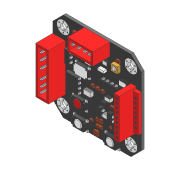
# Autodesk Inventor part: Closed Loop Driver Nema 17
Saved by Autodesk Inventor 2022 (Build 260153000, 153)
## iProperties
Created: 2024-03-01
Part Number: Closed Loop Driver Nema 17
Material: Generic
Document SubType Name: Modeling
Designer: jeffz
Mass: 3.6094 g
Surface Area: 65.104 cm^2
Volume: 3.6094 cm^3
Density: 1 g/cm^3
Appearance: Default
Author: jeffz
Autodesk Inventor part; units mm, degrees
(part 1 of 2)
ref_plane "YZ Plane" through (0, 0, 0) normal (1, 0, 0) x (0, 1, 0)
ref_plane "XZ Plane" through (0, 0, 0) normal (0, 1, 0) x (-1, 0, 0)
ref_plane "XY Plane" through (0, 0, 0) normal (0, 0, 1) x (1, 0, 0)
sketch "Sketch1" plane through (0, 0, 0) normal (0, 0, 1) x (1, 0, 0)
  line L0 (-16, -21) -> (16, -21)
  line L1 (21, -16) -> (21, 16)
  line L2 (16, 21) -> (-16, 21)
  line L3 (-21, 16) -> (-21, -16)
  circle A0 centre (16, 16) radius 1.5
  line L4 (16, 21) -> (21, 16)
  circle A1 centre (16, -16) radius 1.5
  line L5 (21, -16) -> (16, -21)
  circle A2 centre (-16, -16) radius 1.5
  line L6 (-16, -21) -> (-21, -16)
  circle A3 centre (-16, 16) radius 1.5
  line L7 (-21, 16) -> (-16, 21)
  point P0 (0, 0)
  dimension "d2" = 360
  constraints: 16 end point, 4 centre point, 2 parallel, 1 horizontal, 1 perpendicular, 21 other
extrude "Extrusion1" add sketch "Sketch1" along normal blind 1.25
sketch "Sketch2" plane through (0, 0, 1.25) normal (0, 0, 1) x (1, 0, 0)
  circle A0 centre (-16, 16) radius 1.5 projected
  circle A1 centre (-16, -16) radius 1.5 projected
  circle A2 centre (16, -16) radius 1.5 projected
  circle A3 centre (16, 16) radius 1.5 projected
  circle A4 centre (-16, 16) radius 3
  circle A5 centre (-16, 18.2261) radius 0.25
  circle A6 centre (-17.9279, 17.1131) radius 0.25
  circle A7 centre (-17.9279, 14.8869) radius 0.25
  circle A8 centre (-16, 13.7739) radius 0.25
  circle A9 centre (-14.0721, 14.8869) radius 0.25
  circle A10 centre (-14.0721, 17.1131) radius 0.25
  circle A11 centre (-16, -16) radius 3
  circle A12 centre (-16, -13.7739) radius 0.25
  circle A13 centre (-17.9279, -14.8869) radius 0.25
  circle A14 centre (-17.9279, -17.1131) radius 0.25
  circle A15 centre (-16, -18.2261) radius 0.25
  circle A16 centre (-14.0721, -17.1131) radius 0.25
  circle A17 centre (-14.0721, -14.8869) radius 0.25
  circle A18 centre (16, -16) radius 3
  circle A19 centre (16, -13.7739) radius 0.25
  circle A20 centre (14.0721, -14.8869) radius 0.25
  circle A21 centre (14.0721, -17.1131) radius 0.25
  circle A22 centre (16, -18.2261) radius 0.25
  circle A23 centre (17.9279, -17.1131) radius 0.25
  circle A24 centre (17.9279, -14.8869) radius 0.25
  circle A25 centre (16, 16) radius 3
  circle A26 centre (16, 18.2261) radius 0.25
  circle A27 centre (14.0721, 17.1131) radius 0.25
  circle A28 centre (14.0721, 14.8869) radius 0.25
  circle A29 centre (16, 13.7739) radius 0.25
  circle A30 centre (17.9279, 14.8869) radius 0.25
  circle A31 centre (17.9279, 17.1131) radius 0.25
  point P0 (0, 0)
  dimension "d8" = 360
  dimension "d12" = 360
  dimension "d17" = 360
  dimension "d24" = 360
  constraints: 28 centre point, 52 other
extrude "Extrusion2" add sketch "Sketch2" along normal blind 0.05
sketch "Sketch3" plane through (0, 0, 1.25) normal (0, 0, 1) x (1, 0, 0)
  line L0 (-16, -21) -> (16, -21) projected
  line L1 (21, -16) -> (21, 16) projected
  line L2 (16, 21) -> (-16, 21) projected
  line L3 (-21, 16) -> (-21, -16) projected
  line L4 (-21, 11) -> (-15, 11)
  line L5 (-15, 11) -> (-15, -11)
  line L6 (-15, -11) -> (-21, -11)
  line L7 (-21, -11) -> (-21, 11)
  line L8 (-6, 21) -> (6, 21)
  line L9 (6, 21) -> (6, 15)
  line L10 (6, 15) -> (-6, 15)
  line L11 (-6, 15) -> (-6, 21)
  line L12 (18.5, 9) -> (16, 9)
  line L13 (16, 9) -> (16, -10)
  line L14 (16, -10) -> (18.5, -10)
  line L15 (18.5, -10) -> (18.5, 9)
  line L16 (-11, 14) -> (-8, 14)
  line L17 (-8, 14) -> (-8, 11)
  line L18 (-8, 11) -> (-11, 11)
  line L19 (-11, 11) -> (-11, 14)
  line L20 (8, 14) -> (11, 14)
  line L21 (11, 14) -> (11, 11)
  line L22 (11, 11) -> (8, 11)
  line L23 (8, 11) -> (8, 14)
  line L24 (-11, -21) -> (-4, -21)
  line L25 (-4, -21) -> (-4, -16)
  line L26 (-4, -16) -> (-11, -16)
  line L27 (-11, -16) -> (-11, -21)
  line L28 (4, -21) -> (11, -21)
  line L29 (11, -21) -> (11, -16)
  line L30 (11, -16) -> (4, -16)
  line L31 (4, -16) -> (4, -21)
  line L32 (-11.3467, -13) -> (-4.3467, -13)
  line L33 (-4.3467, -13) -> (-4.3467, -8)
  line L34 (-4.3467, -8) -> (-11.3467, -8)
  line L35 (-11.3467, -8) -> (-11.3467, -13)
  line L36 (-10, 1) -> (-3, 1)
  line L37 (-3, 1) -> (-3, 6)
  line L38 (-3, 6) -> (-10, 6)
  line L39 (-10, 6) -> (-10, 1)
  line L40 (-13, 0) -> (-13, -7)
  line L41 (-13, -7) -> (-8, -7)
  line L42 (-8, -7) -> (-8, 0)
  line L43 (-8, 0) -> (-13, 0)
  line L44 (11.7259, -10) -> (15, -10)
  line L45 (15, -10) -> (15, -12)
  line L46 (15, -12) -> (11.7259, -12)
  line L47 (11.7259, -12) -> (11.7259, -10)
  line L48 (11.7259, 9) -> (15, 9)
  line L49 (15, 9) -> (15, 7)
  line L50 (15, 7) -> (11.7259, 7)
  line L51 (11.7259, 7) -> (11.7259, 9)
  line L52 (-6, 13.2927) -> (-4.3467, 13.2927)
  line L53 (-4.3467, 13.2927) -> (-4.3467, 11.7259)
  line L54 (-4.3467, 11.7259) -> (-6, 11.7259)
  line L55 (-6, 11.7259) -> (-6, 13.2927)
  line L56 (-3, 13.2927) -> (-1.3141, 13.2927)
  line L57 (-1.3141, 13.2927) -> (-1.3141, 11.7259)
  line L58 (-1.3141, 11.7259) -> (-3, 11.7259)
  line L59 (-3, 11.7259) -> (-3, 13.2927)
  line L60 (1, 13.2927) -> (2.426, 13.2927)
  line L61 (2.426, 13.2927) -> (2.426, 11.7259)
  line L62 (2.426, 11.7259) -> (1, 11.7259)
  line L63 (1, 11.7259) -> (1, 13.2927)
  line L64 (4, 13.2927) -> (6, 13.2927)
  line L65 (6, 13.2927) -> (6, 11.7259)
  line L66 (6, 11.7259) -> (4, 11.7259)
  line L67 (4, 11.7259) -> (4, 13.2927)
  line L68 (-4.3467, 9) -> (-1.7185, 9)
  line L69 (-1.7185, 9) -> (-1.7185, 8)
  line L70 (-1.7185, 8) -> (-4.3467, 8)
  line L71 (-4.3467, 8) -> (-4.3467, 9)
  line L72 (1.713, 9) -> (4.5488, 9)
  line L73 (4.5488, 9) -> (4.5488, 8)
  line L74 (4.5488, 8) -> (1.713, 8)
  line L75 (1.713, 8) -> (1.713, 9)
  line L76 (18.5, 8) -> (21, 8)
  line L77 (21, 8) -> (21, -9)
  line L78 (21, -9) -> (18.5, -9)
  line L79 (18.5, -9) -> (18.5, 8)
  line L80 (16.861, 8) -> (17.6346, 8)
  line L81 (17.6346, 8) -> (17.6346, 7)
  line L82 (17.6346, 7) -> (16.861, 7)
  line L83 (16.861, 7) -> (16.861, 8)
  line L84 (16.861, 6) -> (17.6346, 6)
  line L85 (17.6346, 6) -> (17.6346, 5)
  line L86 (17.6346, 5) -> (16.861, 5)
  line L87 (16.861, 5) -> (16.861, 6)
  line L88 (16.861, 4) -> (17.6346, 4)
  line L89 (17.6346, 4) -> (17.6346, 3)
  line L90 (17.6346, 3) -> (16.861, 3)
  line L91 (16.861, 3) -> (16.861, 4)
  line L92 (16.8602, 2.1028) -> (17.6337, 2.1028)
  line L93 (17.6337, 2.1028) -> (17.6337, 1.1028)
  line L94 (17.6337, 1.1028) -> (16.8602, 1.1028)
  line L95 (16.8602, 1.1028) -> (16.8602, 2.1028)
  line L96 (16.8602, -0.0613) -> (17.6337, -0.0613)
  line L97 (17.6337, -0.0613) -> (17.6337, -1.0613)
  line L98 (17.6337, -1.0613) -> (16.8602, -1.0613)
  line L99 (16.8602, -1.0613) -> (16.8602, -0.0613)
  line L100 (16.861, -2) -> (17.6346, -2)
  line L101 (17.6346, -2) -> (17.6346, -3)
  line L102 (17.6346, -3) -> (16.861, -3)
  line L103 (16.861, -3) -> (16.861, -2)
  line L104 (16.861, -4) -> (17.6346, -4)
  line L105 (17.6346, -4) -> (17.6346, -5)
  line L106 (17.6346, -5) -> (16.861, -5)
  line L107 (16.861, -5) -> (16.861, -4)
  line L108 (16.861, -6) -> (17.6346, -6)
  line L109 (17.6346, -6) -> (17.6346, -7)
  line L110 (17.6346, -7) -> (16.861, -7)
  line L111 (16.861, -7) -> (16.861, -6)
  line L112 (16.861, -8) -> (17.6346, -8)
  line L113 (17.6346, -8) -> (17.6346, -9)
  line L114 (17.6346, -9) -> (16.861, -9)
  line L115 (16.861, -9) -> (16.861, -8)
  line L116 (-20, 10) -> (-16, 10)
  line L117 (-16, 10) -> (-16, -10)
  line L118 (-16, -10) -> (-20, -10)
  line L119 (-20, -10) -> (-20, 10)
  line L120 (-19, 8.5) -> (-18.3156, 8.5)
  line L121 (-18.3156, 8.5) -> (-18.3156, 8)
  line L122 (-18.3156, 8) -> (-19, 8)
  line L123 (-19, 8) -> (-19, 8.5)
  line L124 (-19, -7.9464) -> (-18.3156, -7.9464)
  line L125 (-18.3156, -7.9464) -> (-18.3156, -8.4464)
  line L126 (-18.3156, -8.4464) -> (-19, -8.4464)
  line L127 (-19, -8.4464) -> (-19, -7.9464)
  line L128 (-19, -5.5) -> (-18.3156, -5.5)
  line L129 (-18.3156, -5.5) -> (-18.3156, -6)
  line L130 (-18.3156, -6) -> (-19, -6)
  line L131 (-19, -6) -> (-19, -5.5)
  line L132 (-19, -2.5) -> (-18.3156, -2.5)
  line L133 (-18.3156, -2.5) -> (-18.3156, -3)
  line L134 (-18.3156, -3) -> (-19, -3)
  line L135 (-19, -3) -> (-19, -2.5)
  line L136 (-19, 1.9327) -> (-18.3156, 1.9327)
  line L137 (-18.3156, 1.9327) -> (-18.3156, 1.4327)
  line L138 (-18.3156, 1.4327) -> (-19, 1.4327)
  line L139 (-19, 1.4327) -> (-19, 1.9327)
  line L140 (-19, 5.3259) -> (-18.3156, 5.3259)
  line L141 (-18.3156, 5.3259) -> (-18.3156, 4.8259)
  line L142 (-18.3156, 4.8259) -> (-19, 4.8259)
  line L143 (-19, 4.8259) -> (-19, 5.3259)
  line L144 (3.1309, -4) -> (5, -4)
  line L145 (5, -4) -> (5, -5)
  line L146 (5, -5) -> (3.1309, -5)
  line L147 (3.1309, -5) -> (3.1309, -4)
  line L148 (5, -1.0613) -> (7.5, -1.0613)
  line L149 (7.5, -1.0613) -> (7.5, -2.5)
  line L150 (7.5, -2.5) -> (5, -2.5)
  line L151 (5, -2.5) -> (5, -1.0613)
  line L152 (2.5, 2.5) -> (11, 2.5)
  line L153 (11, 2.5) -> (11, 4.8259)
  line L154 (11, 4.8259) -> (2.5, 4.8259)
  line L155 (2.5, 4.8259) -> (2.5, 2.5)
  line L156 (6.25, -7) -> (8, -7)
  line L157 (8, -7) -> (8, -11.4558)
  line L158 (8, -11.4558) -> (6.25, -11.4558)
  line L159 (6.25, -11.4558) -> (6.25, -7)
  line L160 (1.713, -7) -> (3.1309, -7)
  line L161 (3.1309, -7) -> (3.1309, -11.4558)
  line L162 (3.1309, -11.4558) -> (1.713, -11.4558)
  line L163 (1.713, -11.4558) -> (1.713, -7)
  line L164 (4.0655, -8.4464) -> (6, -8.4464)
  line L165 (6, -8.4464) -> (6, -10)
  line L166 (6, -10) -> (4.0655, -10)
  line L167 (4.0655, -10) -> (4.0655, -8.4464)
  line L168 (-5.1733, 20) -> (5.0327, 20)
  line L169 (5.0327, 20) -> (5.0327, 16)
  line L170 (5.0327, 16) -> (-5.1733, 16)
  line L171 (-5.1733, 16) -> (-5.1733, 20)
  line L172 (-4.3467, 19) -> (-3.5998, 19)
  line L173 (-3.5998, 19) -> (-3.5998, 18.5)
  line L174 (-3.5998, 18.5) -> (-4.3467, 18.5)
  line L175 (-4.3467, 18.5) -> (-4.3467, 19)
  line L176 (4.5488, 19) -> (3.6544, 19)
  line L177 (3.6544, 19) -> (3.6544, 18.5)
  line L178 (3.6544, 18.5) -> (4.5488, 18.5)
  line L179 (4.5488, 18.5) -> (4.5488, 19)
  line L180 (-1.5055, 19) -> (-0.7289, 19)
  line L181 (-0.7289, 19) -> (-0.7289, 18.5)
  line L182 (-0.7289, 18.5) -> (-1.5055, 18.5)
  line L183 (-1.5055, 18.5) -> (-1.5055, 19)
  line L184 (1.2968, 19) -> (2.1134, 19)
  line L185 (2.1134, 19) -> (2.1134, 18.5)
  line L186 (2.1134, 18.5) -> (1.2968, 18.5)
  line L187 (1.2968, 18.5) -> (1.2968, 19)
  line L188 (20.1465, 5) -> (19.373, 5)
  line L189 (19.373, 5) -> (19.373, 6)
  line L190 (19.373, 6) -> (20.1465, 6)
  line L191 (20.1465, 6) -> (20.1465, 5)
  line L192 (20.1465, 3) -> (19.373, 3)
  line L193 (19.373, 3) -> (19.373, 4)
  line L194 (19.373, 4) -> (20.1465, 4)
  line L195 (20.1465, 4) -> (20.1465, 3)
  line L196 (20.1457, 1.1028) -> (19.3721, 1.1028)
  line L197 (19.3721, 1.1028) -> (19.3721, 2.1028)
  line L198 (19.3721, 2.1028) -> (20.1457, 2.1028)
  line L199 (20.1457, 2.1028) -> (20.1457, 1.1028)
  line L200 (20.1457, -1.0613) -> (19.3721, -1.0613)
  line L201 (19.3721, -1.0613) -> (19.3721, -0.0613)
  line L202 (19.3721, -0.0613) -> (20.1457, -0.0613)
  line L203 (20.1457, -0.0613) -> (20.1457, -1.0613)
  line L204 (20.1465, -3) -> (19.373, -3)
  line L205 (19.373, -3) -> (19.373, -2)
  line L206 (19.373, -2) -> (20.1465, -2)
  line L207 (20.1465, -2) -> (20.1465, -3)
  line L208 (20.1465, -5) -> (19.373, -5)
  line L209 (19.373, -5) -> (19.373, -4)
  line L210 (19.373, -4) -> (20.1465, -4)
  line L211 (20.1465, -4) -> (20.1465, -5)
  line L212 (20.1465, -7) -> (19.373, -7)
  line L213 (19.373, -7) -> (19.373, -6)
  line L214 (19.373, -6) -> (20.1465, -6)
  line L215 (20.1465, -6) -> (20.1465, -7)
  line L216 (-14, 9) -> (-12, 9)
  line L217 (-12, 9) -> (-12, 3)
  line L218 (-12, 3) -> (-14, 3)
  line L219 (-14, 3) -> (-14, 9)
  line L220 (13.3629, -3) -> (11.7259, -3)
  line L221 (11.7259, -3) -> (11.7259, -5.5)
  line L222 (11.7259, -5.5) -> (13.3629, -5.5)
  line L223 (13.3629, -5.5) -> (13.3629, -3)
  line L224 (-5, -3) -> (-1.7185, -3)
  line L225 (-1.7185, -3) -> (-1.7185, -5)
  line L226 (-1.7185, -5) -> (-5, -5)
  line L227 (-5, -5) -> (-5, -3)
  point P0 (0, 0)
  point P1 (21, -9)
  point P2 (6, 21)
  constraints: 448 end point, 112 parallel, 56 perpendicular, 55 horizontal, 31 point on line
extrude "Extrusion3" add sketch "Sketch3" along normal blind 1.5
sketch "Sketch4" plane through (0, 0, 2.75) normal (0, 0, 1) x (1, 0, 0)
  line L0 (-15, 11) -> (-21, 11) projected
  line L1 (-21, 11) -> (-21, -11) projected
  line L2 (-21, -11) -> (-15, -11) projected
  line L3 (-15, -11) -> (-15, 11) projected
  line L4 (-20, 10) -> (-16, 10) projected
  line L5 (-16, 10) -> (-16, -10) projected
  line L6 (-16, -10) -> (-20, -10) projected
  line L7 (-20, -10) -> (-20, 10) projected
  line L8 (-19, 4.8259) -> (-18.3156, 4.8259) projected
  line L9 (-18.3156, 4.8259) -> (-18.3156, 5.3259) projected
  line L10 (-18.3156, 5.3259) -> (-19, 5.3259) projected
  line L11 (-19, 5.3259) -> (-19, 4.8259) projected
  line L12 (-19, 8) -> (-18.3156, 8) projected
  line L13 (-18.3156, 8) -> (-18.3156, 8.5) projected
  line L14 (-18.3156, 8.5) -> (-19, 8.5) projected
  line L15 (-19, 8.5) -> (-19, 8) projected
  line L16 (-19, -7.9464) -> (-19, -8.4464) projected
  line L17 (-19, -8.4464) -> (-18.3156, -8.4464) projected
  line L18 (-18.3156, -8.4464) -> (-18.3156, -7.9464) projected
  line L19 (-18.3156, -7.9464) -> (-19, -7.9464) projected
  line L20 (-19, -7.9464) -> (-19, -8.4464) projected
  line L21 (-18.3156, -5.5) -> (-19, -5.5) projected
  line L22 (-19, -6) -> (-18.3156, -6) projected
  line L23 (-18.3156, -6) -> (-18.3156, -5.5) projected
  line L24 (-18.3156, -5.5) -> (-19, -5.5) projected
  line L25 (-19, -5.5) -> (-19, -6) projected
  line L26 (-19, -3) -> (-18.3156, -3) projected
  line L27 (-18.3156, -3) -> (-18.3156, -2.5) projected
  line L28 (-18.3156, -2.5) -> (-19, -2.5) projected
  line L29 (-19, -2.5) -> (-19, -3) projected
  line L30 (-19, 1.4327) -> (-18.3156, 1.4327) projected
  line L31 (-18.3156, 1.4327) -> (-18.3156, 1.9327) projected
  line L32 (-18.3156, 1.9327) -> (-19, 1.9327) projected
  line L33 (-19, 1.9327) -> (-19, 1.4327) projected
  line L34 (21, -9) -> (21, 8) projected
  line L35 (21, 8) -> (18.5, 8) projected
  line L36 (18.5, 8) -> (18.5, 9) projected
  line L37 (18.5, 9) -> (16, 9) projected
  line L38 (16, 9) -> (16, -10) projected
  line L39 (16, -10) -> (18.5, -10) projected
  line L40 (18.5, -10) -> (18.5, -9) projected
  line L41 (18.5, -9) -> (21, -9) projected
  line L42 (16.861, 8) -> (17.6346, 8) projected
  line L43 (17.6346, 8) -> (17.6346, 7) projected
  line L44 (17.6346, 7) -> (16.861, 7) projected
  line L45 (16.861, 7) -> (16.861, 8) projected
  line L46 (17.6346, 5) -> (16.861, 5) projected
  line L47 (16.861, 5) -> (16.861, 6) projected
  line L48 (16.861, 6) -> (17.6346, 6) projected
  line L49 (17.6346, 6) -> (17.6346, 5) projected
  line L50 (17.6346, 3) -> (16.861, 3) projected
  line L51 (16.861, 3) -> (16.861, 4) projected
  line L52 (16.861, 4) -> (17.6346, 4) projected
  line L53 (17.6346, 4) -> (17.6346, 3) projected
  line L54 (17.6337, 1.1028) -> (16.8602, 1.1028) projected
  line L55 (16.8602, 1.1028) -> (16.8602, 2.1028) projected
  line L56 (16.8602, 2.1028) -> (17.6337, 2.1028) projected
  line L57 (17.6337, 2.1028) -> (17.6337, 1.1028) projected
  line L58 (17.6337, -1.0613) -> (16.8602, -1.0613) projected
  line L59 (16.8602, -1.0613) -> (16.8602, -0.0613) projected
  line L60 (16.8602, -0.0613) -> (17.6337, -0.0613) projected
  line L61 (17.6337, -0.0613) -> (17.6337, -1.0613) projected
  line L62 (17.6346, -3) -> (16.861, -3) projected
  line L63 (16.861, -3) -> (16.861, -2) projected
  line L64 (16.861, -2) -> (17.6346, -2) projected
  line L65 (17.6346, -2) -> (17.6346, -3) projected
  line L66 (17.6346, -5) -> (16.861, -5) projected
  line L67 (16.861, -5) -> (16.861, -4) projected
  line L68 (16.861, -4) -> (17.6346, -4) projected
  line L69 (17.6346, -4) -> (17.6346, -5) projected
  line L70 (17.6346, -7) -> (16.861, -7) projected
  line L71 (16.861, -7) -> (16.861, -6) projected
  line L72 (16.861, -6) -> (17.6346, -6) projected
  line L73 (17.6346, -6) -> (17.6346, -7) projected
  line L74 (17.6346, -9) -> (16.861, -9) projected
  line L75 (16.861, -9) -> (16.861, -8) projected
  line L76 (16.861, -8) -> (17.6346, -8) projected
  line L77 (17.6346, -8) -> (17.6346, -9) projected
  line L78 (20.1465, -7) -> (19.373, -7) projected
  line L79 (19.373, -7) -> (19.373, -6) projected
  line L80 (19.373, -6) -> (20.1465, -6) projected
  line L81 (20.1465, -6) -> (20.1465, -7) projected
  line L82 (19.373, -4) -> (20.1465, -4) projected
  line L83 (20.1465, -4) -> (20.1465, -5) projected
  line L84 (20.1465, -5) -> (19.373, -5) projected
  line L85 (19.373, -5) -> (19.373, -4) projected
  line L86 (19.373, -2) -> (20.1465, -2) projected
  line L87 (20.1465, -2) -> (20.1465, -3) projected
  line L88 (20.1465, -3) -> (19.373, -3) projected
  line L89 (19.373, -3) -> (19.373, -2) projected
  line L90 (20.1465, 5) -> (19.373, 5) projected
  line L91 (19.373, 5) -> (19.373, 6) projected
  line L92 (19.373, 6) -> (20.1465, 6) projected
  line L93 (20.1465, 6) -> (20.1465, 5) projected
  line L94 (19.3721, 2.1028) -> (20.1457, 2.1028) projected
  line L95 (20.1457, 2.1028) -> (20.1457, 1.1028) projected
  line L96 (20.1457, 1.1028) -> (19.3721, 1.1028) projected
  line L97 (19.3721, 1.1028) -> (19.3721, 2.1028) projected
  line L98 (20.1465, 4) -> (20.1465, 3) projected
  line L99 (20.1465, 3) -> (19.373, 3) projected
  line L100 (19.373, 3) -> (19.373, 4) projected
  line L101 (19.373, 4) -> (20.1465, 4) projected
  line L102 (20.1457, -1.0613) -> (19.3721, -1.0613) projected
  line L103 (19.3721, -1.0613) -> (19.3721, -0.0613) projected
  line L104 (19.3721, -0.0613) -> (20.1457, -0.0613) projected
  line L105 (20.1457, -0.0613) -> (20.1457, -1.0613) projected
  line L106 (-11, -16) -> (-11, -21) projected
  line L107 (-11, -21) -> (-4, -21) projected
  line L108 (-4, -21) -> (-4, -16) projected
  line L109 (-4, -16) -> (-11, -16) projected
  line L110 (4, -16) -> (4, -21) projected
  line L111 (4, -21) -> (11, -21) projected
  line L112 (11, -21) -> (11, -16) projected
  line L113 (11, -16) -> (4, -16) projected
  line L114 (-11.3467, -8) -> (-11.3467, -13) projected
  line L115 (-11.3467, -13) -> (-4.3467, -13) projected
  line L116 (-4.3467, -13) -> (-4.3467, -8) projected
  line L117 (-4.3467, -8) -> (-11.3467, -8) projected
  line L118 (-5.1733, 20) -> (-5.1733, 16) projected
  line L119 (-5.1733, 16) -> (5.0327, 16) projected
  line L120 (5.0327, 16) -> (5.0327, 20) projected
  line L121 (5.0327, 20) -> (-5.1733, 20) projected
  line L122 (1.2968, 18.5) -> (1.2968, 19) projected
  line L123 (1.2968, 19) -> (2.1134, 19) projected
  line L124 (2.1134, 19) -> (2.1134, 18.5) projected
  line L125 (2.1134, 18.5) -> (1.2968, 18.5) projected
  line L126 (-4.3467, 18.5) -> (-4.3467, 19) projected
  line L127 (-4.3467, 19) -> (-3.5998, 19) projected
  line L128 (-3.5998, 19) -> (-3.5998, 18.5) projected
  line L129 (-3.5998, 18.5) -> (-4.3467, 18.5) projected
  line L130 (3.6544, 19) -> (4.5488, 19) projected
  line L131 (4.5488, 19) -> (4.5488, 18.5) projected
  line L132 (4.5488, 18.5) -> (3.6544, 18.5) projected
  line L133 (3.6544, 18.5) -> (3.6544, 19) projected
  line L134 (-1.5055, 18.5) -> (-1.5055, 19) projected
  line L135 (-1.5055, 19) -> (-0.7289, 19) projected
  line L136 (-0.7289, 19) -> (-0.7289, 18.5) projected
  line L137 (-0.7289, 18.5) -> (-1.5055, 18.5) projected
  line L138 (6, 15) -> (6, 21) projected
  line L139 (6, 21) -> (-6, 21) projected
  line L140 (-6, 21) -> (-6, 15) projected
  line L141 (-6, 15) -> (6, 15) projected
  line L142 (-5.1733, 20) -> (5.0327, 20) projected
  line L143 (5.0327, 20) -> (5.0327, 16) projected
  line L144 (5.0327, 16) -> (-5.1733, 16) projected
  line L145 (-5.1733, 16) -> (-5.1733, 20) projected
  line L146 (-10, 6) -> (-10, 1) projected
  line L147 (-10, 1) -> (-3, 1) projected
  line L148 (-3, 1) -> (-3, 6) projected
  line L149 (-3, 6) -> (-10, 6) projected
  line L150 (-8, 0) -> (-13, 0) projected
  line L151 (-13, 0) -> (-13, -7) projected
  line L152 (-13, -7) -> (-8, -7) projected
  line L153 (-8, -7) -> (-8, 0) projected
  line L154 (8, 11) -> (11, 11) projected
  line L155 (11, 11) -> (11, 14) projected
  line L156 (11, 14) -> (8, 14) projected
  line L157 (8, 14) -> (8, 11) projected
  line L158 (-11, 11) -> (-8, 11) projected
  line L159 (-8, 11) -> (-8, 14) projected
  line L160 (-8, 14) -> (-11, 14) projected
  line L161 (-11, 14) -> (-11, 11) projected
  point P0 (0, 0)
extrude "Extrusion4" add sketch "Sketch4" along normal blind 1
sketch "Sketch5" plane through (0, 0, 3.75) normal (0, 0, 1) x (1, 0, 0)
  line L0 (-4, -21) -> (-4, -16) projected
  line L1 (-4, -16) -> (-11, -16) projected
  line L2 (-11, -16) -> (-11, -21) projected
  line L3 (-11.3467, -13) -> (-4.3467, -13) projected
  line L4 (-4.3467, -13) -> (-4.3467, -8) projected
  line L5 (-4.3467, -8) -> (-11.3467, -8) projected
  line L6 (-11.3467, -8) -> (-11.3467, -13) projected
  line L7 (4, -21) -> (11, -21) projected
  line L8 (11, -21) -> (11, -16) projected
  line L9 (11, -16) -> (4, -16) projected
  line L10 (4, -16) -> (4, -21) projected
  circle A0 centre (-7.5, -18.5) radius 1.9305
  circle A1 centre (7.5, -18.5) radius 1.9305
  circle A2 centre (-7.8467, -10.5) radius 1.9305
  line L11 (-8, 11) -> (-8, 14) projected
  line L12 (-8, 14) -> (-11, 14) projected
  line L13 (-11, 14) -> (-11, 11) projected
  line L14 (-11, 11) -> (-8, 11) projected
  line L15 (11, 11) -> (11, 14) projected
  line L16 (11, 14) -> (8, 14) projected
  line L17 (8, 14) -> (8, 11) projected
  line L18 (8, 11) -> (11, 11) projected
  circle A3 centre (-9.5, 12.5) radius 1.2112
  circle A4 centre (9.5, 12.5) radius 1.2112
  line L19 (-11, -21) -> (-11, -16) projected
  line L20 (-11, -17) -> (-10.7112, -17)
  line L21 (-10.7112, -17) -> (-10.7112, -20)
  line L22 (-10.7112, -20) -> (-11, -20)
  line L23 (-11, -20) -> (-11, -17)
  line L24 (-11.3467, -9) -> (-11.0579, -9)
  line L25 (-11.0579, -9) -> (-11.0579, -12)
  line L26 (-11.0579, -12) -> (-11.3467, -12)
  line L27 (-11.3467, -12) -> (-11.3467, -9)
  line L28 (4, -17) -> (4.2888, -17)
  line L29 (4.2888, -17) -> (4.2888, -20)
  line L30 (4.2888, -20) -> (4, -20)
  line L31 (4, -20) -> (4, -17)
  line L32 (-10.7112, -17) -> (-10.7112, -16)
  line L33 (-11, -16) -> (-4, -16) projected
  line L34 (-4.2888, -17) -> (-4, -17)
  line L35 (-4, -17) -> (-4, -20)
  line L36 (-4, -20) -> (-4.2888, -20)
  line L37 (-4.2888, -20) -> (-4.2888, -17)
  line L38 (-4, -17) -> (-4, -16)
  line L39 (10.7112, -17) -> (11, -17)
  line L40 (11, -17) -> (11, -20)
  line L41 (11, -20) -> (10.7112, -20)
  line L42 (10.7112, -20) -> (10.7112, -17)
  line L43 (11, -17) -> (11, -16)
  line L44 (-4.6355, -9) -> (-4.3467, -9)
  line L45 (-4.3467, -9) -> (-4.3467, -12)
  line L46 (-4.3467, -12) -> (-4.6355, -12)
  line L47 (-4.6355, -12) -> (-4.6355, -9)
  line L48 (-4.3467, -9) -> (-4.3467, -8)
  line L49 (-10, 1) -> (-3, 1) projected
  line L50 (-3, 1) -> (-3, 6) projected
  line L51 (-3, 6) -> (-10, 6) projected
  line L52 (-10, 6) -> (-10, 1) projected
  line L53 (-13, 0) -> (-13, -7) projected
  line L54 (-13, -7) -> (-8, -7) projected
  line L55 (-8, -7) -> (-8, 0) projected
  line L56 (-8, 0) -> (-13, 0) projected
  line L57 (-3, 5) -> (-3, 6)
  line L58 (-3.2888, 5) -> (-3, 5)
  line L59 (-3, 5) -> (-3, 2)
  line L60 (-3, 2) -> (-3.2888, 2)
  line L61 (-3.2888, 2) -> (-3.2888, 5)
  line L62 (-9.7112, 5) -> (-9.7112, 2)
  line L63 (-9.7112, 2) -> (-10, 2)
  line L64 (-10, 5) -> (-9.7112, 5)
  line L65 (-10, 2) -> (-10, 5)
  point P0 (0, 0)
  constraints: 74 end point, 16 parallel, 9 perpendicular, 8 horizontal, 5 centre point, 2 point on line
extrude "Extrusion5" cut sketch "Sketch5" against normal up to surface (2.5 mm away) contours L36 L37 L34 L0 | L21 L22 L2 L20 | L6 L24 L25 L26 | L46 L47 L44 L4 | L10 L28 L29 L30 | L41 L42 L39 L8 | L52 L64 L62 L63 | L60 L61 L58 L50
sketch "Sketch6" plane through (0, 0, 3.75) normal (0, 0, 1) x (1, 0, 0)
  line L0 (-4, -16) -> (-11, -16) projected
  line L1 (-11, -21) -> (-4, -21) projected
  line L2 (-10, 5) -> (-9.7112, 5) projected
  line L3 (-9.7112, 5) -> (-9.7112, 2) projected
  line L4 (-9.7112, 2) -> (-10, 2) projected
  line L5 (-10, 2) -> (-10, 1) projected
  line L6 (-10, 1) -> (-3, 1) projected
  line L7 (-3, 1) -> (-3, 2) projected
  line L8 (-3, 2) -> (-3.2888, 2) projected
  line L9 (-3.2888, 2) -> (-3.2888, 5) projected
  line L10 (-3.2888, 5) -> (-3, 5) projected
  line L11 (-3, 5) -> (-3, 6) projected
  line L12 (-3, 6) -> (-10, 6) projected
  line L13 (-10, 6) -> (-10, 5) projected
  line L14 (-4.3467, -12) -> (-4.6355, -12) projected
  line L15 (-4.6355, -12) -> (-4.6355, -9) projected
  line L16 (-4.6355, -9) -> (-4.3467, -9) projected
  line L17 (-4.3467, -9) -> (-4.3467, -8) projected
  line L18 (-4.3467, -8) -> (-11.3467, -8) projected
  line L19 (-11.3467, -8) -> (-11.3467, -9) projected
  line L20 (-11.3467, -9) -> (-11.0579, -9) projected
  line L21 (-11.0579, -9) -> (-11.0579, -12) projected
  line L22 (-11.0579, -12) -> (-11.3467, -12) projected
  line L23 (-11.3467, -12) -> (-11.3467, -13) projected
  line L24 (-11.3467, -13) -> (-4.3467, -13) projected
  line L25 (-4.3467, -13) -> (-4.3467, -12) projected
  line L26 (4, -17) -> (4.2888, -17) projected
  line L27 (4.2888, -17) -> (4.2888, -20) projected
  line L28 (4.2888, -20) -> (4, -20) projected
  line L29 (4, -20) -> (4, -21) projected
  line L30 (4, -21) -> (11, -21) projected
  line L31 (11, -21) -> (11, -20) projected
  line L32 (11, -20) -> (10.7112, -20) projected
  line L33 (10.7112, -20) -> (10.7112, -17) projected
  line L34 (10.7112, -17) -> (11, -17) projected
  line L35 (11, -17) -> (11, -16) projected
  line L36 (11, -16) -> (4, -16) projected
  line L37 (4, -16) -> (4, -17) projected
  line L38 (11, 11) -> (11, 14) projected
  line L39 (11, 14) -> (8, 14) projected
  line L40 (8, 14) -> (8, 11) projected
  line L41 (8, 11) -> (11, 11) projected
  line L42 (-8, 11) -> (-8, 14) projected
  line L43 (-8, 14) -> (-11, 14) projected
  line L44 (-11, 14) -> (-11, 11) projected
  line L45 (-11, 11) -> (-8, 11) projected
  circle A0 centre (-7.5, -18.5) radius 1.9686
  line L46 (-8, -10.5) -> (-7.8467, -10.5)
  circle A1 centre (-7.8467, -10.5) radius 1.9686
  circle A2 centre (7.5, -18.5) radius 1.9686
  line L47 (-10, 6) -> (-3, 6) projected
  line L48 (-9, 6) -> (-4, 6)
  line L49 (-4, 6) -> (-4, 5.75)
  line L50 (-4, 5.75) -> (-9, 5.75)
  line L51 (-9, 5.75) -> (-9, 6)
  line L52 (11, -16) -> (4, -16) projected
  line L53 (-4.3467, -8) -> (-11.3467, -8) projected
  line L54 (-5.3467, -8.25) -> (-10.3467, -8.25)
  line L55 (-10.3467, -8) -> (-5.3467, -8)
  line L56 (-10.3467, -8.25) -> (-10.3467, -8)
  line L57 (-5.3467, -8) -> (-5.3467, -8.25)
  line L58 (-5, -16.25) -> (-10, -16.25)
  line L59 (-10, -16) -> (-5, -16)
  line L60 (-10, -16.25) -> (-10, -16)
  line L61 (-5, -16) -> (-5, -16.25)
  line L62 (10, -16.25) -> (5, -16.25)
  line L63 (5, -16) -> (10, -16)
  line L64 (5, -16.25) -> (5, -16)
  line L65 (10, -16) -> (10, -16.25)
  line L66 (-10, 1) -> (-3, 1) projected
  line L67 (-11.3467, -13) -> (-4.3467, -13) projected
  line L68 (4, -21) -> (11, -21) projected
  line L69 (-4, 1) -> (-9, 1)
  line L70 (-9, 1.25) -> (-4, 1.25)
  line L71 (-9, 1) -> (-9, 1.25)
  line L72 (-4, 1.25) -> (-4, 1)
  line L73 (-5.3467, -13) -> (-10.3467, -13)
  line L74 (-10.3467, -12.75) -> (-5.3467, -12.75)
  line L75 (-10.3467, -13) -> (-10.3467, -12.75)
  line L76 (-5.3467, -12.75) -> (-5.3467, -13)
  line L77 (-5, -21) -> (-10, -21)
  line L78 (-10, -20.75) -> (-5, -20.75)
  line L79 (-10, -21) -> (-10, -20.75)
  line L80 (-5, -20.75) -> (-5, -21)
  line L81 (10, -21) -> (5, -21)
  line L82 (5, -20.75) -> (10, -20.75)
  line L83 (5, -21) -> (5, -20.75)
  line L84 (10, -20.75) -> (10, -21)
  circle A3 centre (-9.4686, 12.5) radius 1.0483
  circle A4 centre (9.4686, 12.5) radius 1.0483
  point P0 (0, 0)
  constraints: 66 end point, 16 parallel, 8 horizontal, 8 perpendicular, 5 centre point, 1 point on line
extrude "Extrusion6" cut sketch "Sketch6" against normal up to surface (2.5 mm away) contours L61 L58 L60 L0 | L79 L78 L80 L1 | L12 L49 L50 L51 | L71 L70 L72 L6 | L24 L75 L74 L76 | L57 L54 L56 L18 | L36 L65 L62 L64 | L83 L82 L84 L30 | A0 | A1 | A2 | A3 | A4
sketch "Sketch7" plane through (-7.8467, -10.5, 1.25) normal (0, 0, 1) x (1, 0, 0)
  circle A0 centre (0, 0) radius 1.9686 projected
  circle A1 centre (15.3467, -8) radius 1.9686 projected
  circle A2 centre (0.3467, -8) radius 1.9686 projected
  circle A3 centre (17.3153, 23) radius 1.0483 projected
  circle A4 centre (-1.622, 23) radius 1.0483 projected
  circle A5 centre (-1.622, 23) radius 0.9233
  circle A6 centre (17.3153, 23) radius 0.9233
  circle A7 centre (0, 0) radius 2.0936
  circle A8 centre (0, 0) radius 1.843
  circle A9 centre (15.3467, -8) radius 1.8436
  circle A10 centre (0.3467, -8) radius 1.8436
  line L0 (-2.1533, -5.75) -> (-2.1533, -5.5) projected
  line L1 (-2.1533, -5.5) -> (-3.1533, -5.5) projected
  line L2 (-3.1533, -5.5) -> (-3.1533, -6.5) projected
  line L3 (-3.1533, -6.5) -> (-2.8645, -6.5) projected
  line L4 (-2.8645, -6.5) -> (-2.8645, -9.5) projected
  line L5 (-2.8645, -9.5) -> (-3.1533, -9.5) projected
  line L6 (-3.1533, -9.5) -> (-3.1533, -10.5) projected
  line L7 (-3.1533, -10.5) -> (-2.1533, -10.5) projected
  line L8 (-2.1533, -10.5) -> (-2.1533, -10.25) projected
  line L9 (-2.1533, -10.25) -> (2.8467, -10.25) projected
  line L10 (2.8467, -10.25) -> (2.8467, -10.5) projected
  line L11 (2.8467, -10.5) -> (3.8467, -10.5) projected
  line L12 (3.8467, -10.5) -> (3.8467, -9.5) projected
  line L13 (3.8467, -9.5) -> (3.5579, -9.5) projected
  line L14 (3.5579, -9.5) -> (3.5579, -6.5) projected
  line L15 (3.5579, -6.5) -> (3.8467, -6.5) projected
  line L16 (3.8467, -6.5) -> (3.8467, -5.5) projected
  line L17 (3.8467, -5.5) -> (2.8467, -5.5) projected
  line L18 (2.8467, -5.5) -> (2.8467, -5.75) projected
  line L19 (2.8467, -5.75) -> (-2.1533, -5.75) projected
  circle A11 centre (0.3467, -8) radius 1.9686 projected
  line L20 (18.8467, -5.5) -> (18.8467, -10.5) projected
  line L21 (18.8467, -10.5) -> (23.8467, -10.5) projected
  line L22 (23.8467, -10.5) -> (28.8467, -5.5) projected
  line L23 (28.8467, -5.5) -> (28.8467, 1.5) projected
  line L24 (28.8467, 1.5) -> (26.3467, 1.5) projected
  line L25 (26.3467, 1.5) -> (26.3467, 0.5) projected
  line L26 (26.3467, 0.5) -> (23.8467, 0.5) projected
  line L27 (23.8467, 0.5) -> (23.8467, 19.5) projected
  line L28 (23.8467, 19.5) -> (26.3467, 19.5) projected
  line L29 (26.3467, 19.5) -> (26.3467, 18.5) projected
  line L30 (26.3467, 18.5) -> (28.8467, 18.5) projected
  line L31 (28.8467, 18.5) -> (28.8467, 26.5) projected
  line L32 (28.8467, 26.5) -> (23.8467, 31.5) projected
  line L33 (23.8467, 31.5) -> (13.8467, 31.5) projected
  line L34 (13.8467, 31.5) -> (13.8467, 25.5) projected
  line L35 (13.8467, 25.5) -> (1.8467, 25.5) projected
  line L36 (1.8467, 25.5) -> (1.8467, 31.5) projected
  line L37 (1.8467, 31.5) -> (-8.1533, 31.5) projected
  line L38 (-8.1533, 31.5) -> (-13.1533, 26.5) projected
  line L39 (-13.1533, 26.5) -> (-13.1533, 21.5) projected
  line L40 (-13.1533, 21.5) -> (-7.1533, 21.5) projected
  line L41 (-7.1533, 21.5) -> (-7.1533, -0.5) projected
  line L42 (-7.1533, -0.5) -> (-13.1533, -0.5) projected
  line L43 (-13.1533, -0.5) -> (-13.1533, -5.5) projected
  line L44 (-13.1533, -5.5) -> (-8.1533, -10.5) projected
  line L45 (-8.1533, -10.5) -> (-3.1533, -10.5) projected
  line L46 (-3.1533, -10.5) -> (-3.1533, -5.5) projected
  line L47 (-3.1533, -5.5) -> (-2.1533, -5.5) projected
  line L48 (-2.1533, -5.75) -> (-2.1533, -5.5) projected
  line L49 (2.8467, -5.75) -> (-2.1533, -5.75) projected
  line L50 (2.8467, -5.5) -> (2.8467, -5.75) projected
  line L51 (2.8467, -5.5) -> (3.8467, -5.5) projected
  line L52 (3.8467, -5.5) -> (3.8467, -10.5) projected
  line L53 (3.8467, -10.5) -> (11.8467, -10.5) projected
  line L54 (11.8467, -10.5) -> (11.8467, -5.5) projected
  line L55 (11.8467, -5.5) -> (12.8467, -5.5) projected
  line L56 (12.8467, -5.75) -> (12.8467, -5.5) projected
  line L57 (17.8467, -5.75) -> (12.8467, -5.75) projected
  line L58 (17.8467, -5.5) -> (17.8467, -5.75) projected
  line L59 (17.8467, -5.5) -> (18.8467, -5.5) projected
  line L60 (8.8467, 22.2259) -> (8.8467, 23.7927) projected
  line L61 (8.8467, 23.7927) -> (10.2727, 23.7927) projected
  line L62 (10.2727, 23.7927) -> (10.2727, 22.2259) projected
  line L63 (10.2727, 22.2259) -> (8.8467, 22.2259) projected
  line L64 (12.8467, 8) -> (12.8467, 9.4387) projected
  line L65 (12.8467, 9.4387) -> (15.3467, 9.4387) projected
  line L66 (15.3467, 9.4387) -> (15.3467, 8) projected
  line L67 (15.3467, 8) -> (12.8467, 8) projected
  line L68 (11.9121, 0.5) -> (11.9121, 2.0536) projected
  line L69 (11.9121, 2.0536) -> (13.8467, 2.0536) projected
  line L70 (13.8467, 2.0536) -> (13.8467, 0.5) projected
  line L71 (13.8467, 0.5) -> (11.9121, 0.5) projected
  line L72 (-2.1533, 16.5) -> (-1.1533, 16.5) projected
  line L73 (-1.1533, 16.25) -> (-1.1533, 16.5) projected
  line L74 (3.8467, 16.25) -> (-1.1533, 16.25) projected
  line L75 (3.8467, 16.5) -> (3.8467, 16.25) projected
  line L76 (3.8467, 16.5) -> (4.8467, 16.5) projected
  line L77 (4.8467, 16.5) -> (4.8467, 11.5) projected
  line L78 (4.8467, 11.5) -> (3.8467, 11.5) projected
  line L79 (3.8467, 11.75) -> (3.8467, 11.5) projected
  line L80 (-1.1533, 11.75) -> (3.8467, 11.75) projected
  line L81 (-1.1533, 11.5) -> (-1.1533, 11.75) projected
  line L82 (-1.1533, 11.5) -> (-2.1533, 11.5) projected
  line L83 (-2.1533, 11.5) -> (-2.1533, 16.5) projected
  line L84 (3.5, 18.5) -> (3.5, 19.5) projected
  line L85 (3.5, 19.5) -> (6.1282, 19.5) projected
  line L86 (6.1282, 19.5) -> (6.1282, 18.5) projected
  line L87 (6.1282, 18.5) -> (3.5, 18.5) projected
  line L88 (-6.1533, 13.5) -> (-6.1533, 19.5) projected
  line L89 (-6.1533, 19.5) -> (-4.1533, 19.5) projected
  line L90 (-4.1533, 19.5) -> (-4.1533, 13.5) projected
  line L91 (-4.1533, 13.5) -> (-6.1533, 13.5) projected
  line L92 (-0.1533, 10.5) -> (-0.1533, 3.5) projected
  line L93 (-0.1533, 3.5) -> (-5.1533, 3.5) projected
  line L94 (-5.1533, 3.5) -> (-5.1533, 10.5) projected
  line L95 (-5.1533, 10.5) -> (-0.1533, 10.5) projected
  line L96 (18.8467, 13) -> (10.3467, 13) projected
  line L97 (10.3467, 13) -> (10.3467, 15.3259) projected
  line L98 (10.3467, 15.3259) -> (18.8467, 15.3259) projected
  line L99 (18.8467, 15.3259) -> (18.8467, 13) projected
  line L100 (11.8467, 22.2259) -> (11.8467, 23.7927) projected
  line L101 (11.8467, 23.7927) -> (13.8467, 23.7927) projected
  line L102 (13.8467, 23.7927) -> (13.8467, 22.2259) projected
  line L103 (13.8467, 22.2259) -> (11.8467, 22.2259) projected
  line L104 (15.8467, 21.5) -> (15.8467, 24.5) projected
  line L105 (15.8467, 24.5) -> (18.8467, 24.5) projected
  line L106 (18.8467, 24.5) -> (18.8467, 21.5) projected
  line L107 (18.8467, 21.5) -> (15.8467, 21.5) projected
  line L108 (19.5726, 17.5) -> (19.5726, 19.5) projected
  line L109 (19.5726, 19.5) -> (22.8467, 19.5) projected
  line L110 (22.8467, 19.5) -> (22.8467, 17.5) projected
  line L111 (22.8467, 17.5) -> (19.5726, 17.5) projected
  line L112 (10.9776, 5.5) -> (10.9776, 6.5) projected
  line L113 (10.9776, 6.5) -> (12.8467, 6.5) projected
  line L114 (12.8467, 6.5) -> (12.8467, 5.5) projected
  line L115 (12.8467, 5.5) -> (10.9776, 5.5) projected
  line L116 (9.5597, -0.9558) -> (9.5597, 3.5) projected
  line L117 (9.5597, 3.5) -> (10.9776, 3.5) projected
  line L118 (10.9776, 3.5) -> (10.9776, -0.9558) projected
  line L119 (10.9776, -0.9558) -> (9.5597, -0.9558) projected
  line L120 (19.5726, 7.5) -> (21.2096, 7.5) projected
  line L121 (21.2096, 7.5) -> (21.2096, 5) projected
  line L122 (21.2096, 5) -> (19.5726, 5) projected
  line L123 (19.5726, 5) -> (19.5726, 7.5) projected
  line L124 (-3.5, 2.5) -> (-2.5, 2.5) projected
  line L125 (-2.5, 2.25) -> (-2.5, 2.5) projected
  line L126 (2.5, 2.25) -> (-2.5, 2.25) projected
  line L127 (2.5, 2.5) -> (2.5, 2.25) projected
  line L128 (2.5, 2.5) -> (3.5, 2.5) projected
  line L129 (3.5, 2.5) -> (3.5, -2.5) projected
  line L130 (3.5, -2.5) -> (2.5, -2.5) projected
  line L131 (2.5, -2.25) -> (2.5, -2.5) projected
  line L132 (-2.5, -2.25) -> (2.5, -2.25) projected
  line L133 (-2.5, -2.5) -> (-2.5, -2.25) projected
  line L134 (-2.5, -2.5) -> (-3.5, -2.5) projected
  line L135 (-3.5, -2.5) -> (-3.5, 2.5) projected
  line L136 (4.8467, 22.2259) -> (4.8467, 23.7927) projected
  line L137 (4.8467, 23.7927) -> (6.5326, 23.7927) projected
  line L138 (6.5326, 23.7927) -> (6.5326, 22.2259) projected
  line L139 (6.5326, 22.2259) -> (4.8467, 22.2259) projected
  line L140 (2.8467, 5.5) -> (2.8467, 7.5) projected
  line L141 (2.8467, 7.5) -> (6.1282, 7.5) projected
  line L142 (6.1282, 7.5) -> (6.1282, 5.5) projected
  line L143 (6.1282, 5.5) -> (2.8467, 5.5) projected
  line L144 (1.8467, 22.2259) -> (1.8467, 23.7927) projected
  line L145 (1.8467, 23.7927) -> (3.5, 23.7927) projected
  line L146 (3.5, 23.7927) -> (3.5, 22.2259) projected
  line L147 (3.5, 22.2259) -> (1.8467, 22.2259) projected
  line L148 (-3.1533, 21.5) -> (-3.1533, 24.5) projected
  line L149 (-3.1533, 24.5) -> (-0.1533, 24.5) projected
  line L150 (-0.1533, 24.5) -> (-0.1533, 21.5) projected
  line L151 (-0.1533, 21.5) -> (-3.1533, 21.5) projected
  line L152 (14.0967, -0.9558) -> (14.0967, 3.5) projected
  line L153 (14.0967, 3.5) -> (15.8467, 3.5) projected
  line L154 (15.8467, 3.5) -> (15.8467, -0.9558) projected
  line L155 (15.8467, -0.9558) -> (14.0967, -0.9558) projected
  line L156 (9.5597, 18.5) -> (9.5597, 19.5) projected
  line L157 (9.5597, 19.5) -> (12.3955, 19.5) projected
  line L158 (12.3955, 19.5) -> (12.3955, 18.5) projected
  line L159 (12.3955, 18.5) -> (9.5597, 18.5) projected
  line L160 (19.5726, -1.5) -> (19.5726, 0.5) projected
  line L161 (19.5726, 0.5) -> (22.8467, 0.5) projected
  line L162 (22.8467, 0.5) -> (22.8467, -1.5) projected
  line L163 (22.8467, -1.5) -> (19.5726, -1.5) projected
  circle A12 centre (23.8467, -5.5) radius 3 projected
  circle A13 centre (23.8467, 26.5) radius 3 projected
  circle A14 centre (-8.1533, -5.5) radius 3 projected
  circle A15 centre (-8.1533, 26.5) radius 3 projected
  point P0 (7.8467, 10.5)
  constraints: 6 centre point
extrude "Extrusion7" add sketch "Sketch7" along normal blind 1.75 contours A5 | A6 | A8 | A9 | A10
sketch "Sketch8" plane through (0, 0, 3.75) normal (0, 0, 1) x (1, 0, 0)
  line L0 (-10, -21) -> (-10, -20.75)
  line L1 (-10, -20.75) -> (-5, -20.75)
  line L2 (-5, -20.75) -> (-5, -21)
  line L3 (-5, -21) -> (-4, -21)
  line L4 (-4, -21) -> (-4, -20)
  line L5 (-4, -20) -> (-4.2888, -20)
  line L6 (-4.2888, -20) -> (-4.2888, -17)
  line L7 (-4.2888, -17) -> (-4, -17)
  line L8 (-4, -17) -> (-4, -16)
  line L9 (-4, -16) -> (-5, -16)
  line L10 (-5, -16) -> (-5, -16.25)
  line L11 (-5, -16.25) -> (-10, -16.25)
  line L12 (-10, -16.25) -> (-10, -16)
  line L13 (-10, -16) -> (-11, -16)
  line L14 (-11, -16) -> (-11, -17)
  line L15 (-11, -17) -> (-10.7112, -17)
  line L16 (-10.7112, -17) -> (-10.7112, -20)
  line L17 (-10.7112, -20) -> (-11, -20)
  line L18 (-11, -20) -> (-11, -21)
  line L19 (-11, -21) -> (-10, -21)
  circle A0 centre (-7.5, -18.5) radius 1.9686
  line L20 (10, -16) -> (10, -16.25)
  line L21 (10, -16.25) -> (5, -16.25)
  line L22 (5, -16.25) -> (5, -16)
  line L23 (5, -16) -> (4, -16)
  line L24 (4, -16) -> (4, -17)
  line L25 (4, -17) -> (4.2888, -17)
  line L26 (4.2888, -17) -> (4.2888, -20)
  line L27 (4.2888, -20) -> (4, -20)
  line L28 (4, -20) -> (4, -21)
  line L29 (4, -21) -> (5, -21)
  line L30 (5, -21) -> (5, -20.75)
  line L31 (5, -20.75) -> (10, -20.75)
  line L32 (10, -20.75) -> (10, -21)
  line L33 (10, -21) -> (11, -21)
  line L34 (11, -21) -> (11, -20)
  line L35 (11, -20) -> (10.7112, -20)
  line L36 (10.7112, -20) -> (10.7112, -17)
  line L37 (10.7112, -17) -> (11, -17)
  line L38 (11, -17) -> (11, -16)
  line L39 (11, -16) -> (10, -16)
  circle A1 centre (7.5, -18.5) radius 1.9686
  line L40 (-10.3467, -13) -> (-10.3467, -12.75)
  line L41 (-10.3467, -12.75) -> (-5.3467, -12.75)
  line L42 (-5.3467, -12.75) -> (-5.3467, -13)
  line L43 (-5.3467, -13) -> (-4.3467, -13)
  line L44 (-4.3467, -13) -> (-4.3467, -12)
  line L45 (-4.3467, -12) -> (-4.6355, -12)
  line L46 (-4.6355, -12) -> (-4.6355, -9)
  line L47 (-4.6355, -9) -> (-4.3467, -9)
  line L48 (-4.3467, -9) -> (-4.3467, -8)
  line L49 (-4.3467, -8) -> (-5.3467, -8)
  line L50 (-5.3467, -8) -> (-5.3467, -8.25)
  line L51 (-5.3467, -8.25) -> (-10.3467, -8.25)
  line L52 (-10.3467, -8.25) -> (-10.3467, -8)
  line L53 (-10.3467, -8) -> (-11.3467, -8)
  line L54 (-11.3467, -8) -> (-11.3467, -9)
  line L55 (-11.3467, -9) -> (-11.0579, -9)
  line L56 (-11.0579, -9) -> (-11.0579, -12)
  line L57 (-11.0579, -12) -> (-11.3467, -12)
  line L58 (-11.3467, -12) -> (-11.3467, -13)
  line L59 (-11.3467, -13) -> (-10.3467, -13)
  circle A2 centre (-7.8467, -10.5) radius 1.9686
  circle A3 centre (9.4686, 12.5) radius 1.0483
  line L60 (11, 11) -> (11, 14)
  line L61 (11, 14) -> (8, 14)
  line L62 (8, 14) -> (8, 11)
  line L63 (8, 11) -> (11, 11)
  circle A4 centre (-9.4686, 12.5) radius 1.0483
  line L64 (-8, 11) -> (-8, 14)
  line L65 (-8, 14) -> (-11, 14)
  line L66 (-11, 14) -> (-11, 11)
  line L67 (-11, 11) -> (-8, 11)
  line L68 (-13, 0) -> (-13, -7)
  line L69 (-13, -7) -> (-8, -7)
  line L70 (-8, -7) -> (-8, 0)
  line L71 (-8, 0) -> (-13, 0)
  line L72 (-4, 6) -> (-4, 5.75)
  line L73 (-4, 5.75) -> (-9, 5.75)
  line L74 (-9, 5.75) -> (-9, 6)
  line L75 (-9, 6) -> (-10, 6)
  line L76 (-10, 6) -> (-10, 5)
  line L77 (-10, 5) -> (-9.7112, 5)
  line L78 (-9.7112, 5) -> (-9.7112, 2)
  line L79 (-9.7112, 2) -> (-10, 2)
  line L80 (-10, 2) -> (-10, 1)
  line L81 (-10, 1) -> (-9, 1)
  line L82 (-9, 1) -> (-9, 1.25)
  line L83 (-9, 1.25) -> (-4, 1.25)
  line L84 (-4, 1.25) -> (-4, 1)
  line L85 (-4, 1) -> (-3, 1)
  line L86 (-3, 1) -> (-3, 2)
  line L87 (-3, 2) -> (-3.2888, 2)
  line L88 (-3.2888, 2) -> (-3.2888, 5)
  line L89 (-3.2888, 5) -> (-3, 5)
  line L90 (-3, 5) -> (-3, 6)
  line L91 (-3, 6) -> (-4, 6)
  line L92 (21, 8) -> (18.5, 8)
  line L93 (18.5, 8) -> (18.5, 9)
  line L94 (18.5, 9) -> (16, 9)
  line L95 (16, 9) -> (16, -10)
  line L96 (16, -10) -> (18.5, -10)
  line L97 (18.5, -10) -> (18.5, -9)
  line L98 (18.5, -9) -> (21, -9)
  line L99 (21, -9) -> (21, 8)
  line L100 (20.1457, -1.0613) -> (19.3721, -1.0613)
  line L101 (19.3721, -1.0613) -> (19.3721, -0.0613)
  line L102 (19.3721, -0.0613) -> (20.1457, -0.0613)
  line L103 (20.1457, -0.0613) -> (20.1457, -1.0613)
  line L104 (20.1465, 4) -> (20.1465, 3)
  line L105 (20.1465, 3) -> (19.373, 3)
  line L106 (19.373, 3) -> (19.373, 4)
  line L107 (19.373, 4) -> (20.1465, 4)
  line L108 (19.3721, 2.1028) -> (20.1457, 2.1028)
  line L109 (20.1457, 2.1028) -> (20.1457, 1.1028)
  line L110 (20.1457, 1.1028) -> (19.3721, 1.1028)
  line L111 (19.3721, 1.1028) -> (19.3721, 2.1028)
  line L112 (20.1465, 5) -> (19.373, 5)
  line L113 (19.373, 5) -> (19.373, 6)
  line L114 (19.373, 6) -> (20.1465, 6)
  line L115 (20.1465, 6) -> (20.1465, 5)
  line L116 (19.373, -2) -> (20.1465, -2)
  line L117 (20.1465, -2) -> (20.1465, -3)
  line L118 (20.1465, -3) -> (19.373, -3)
  line L119 (19.373, -3) -> (19.373, -2)
  line L120 (19.373, -4) -> (20.1465, -4)
  line L121 (20.1465, -4) -> (20.1465, -5)
  line L122 (20.1465, -5) -> (19.373, -5)
  line L123 (19.373, -5) -> (19.373, -4)
  line L124 (20.1465, -7) -> (19.373, -7)
  line L125 (19.373, -7) -> (19.373, -6)
  line L126 (19.373, -6) -> (20.1465, -6)
  line L127 (20.1465, -6) -> (20.1465, -7)
  line L128 (17.6346, -9) -> (16.861, -9)
  line L129 (16.861, -9) -> (16.861, -8)
  line L130 (16.861, -8) -> (17.6346, -8)
  line L131 (17.6346, -8) -> (17.6346, -9)
  line L132 (17.6346, -7) -> (16.861, -7)
  line L133 (16.861, -7) -> (16.861, -6)
  line L134 (16.861, -6) -> (17.6346, -6)
  line L135 (17.6346, -6) -> (17.6346, -7)
  line L136 (17.6346, -5) -> (16.861, -5)
  line L137 (16.861, -5) -> (16.861, -4)
  line L138 (16.861, -4) -> (17.6346, -4)
  line L139 (17.6346, -4) -> (17.6346, -5)
  line L140 (17.6346, -3) -> (16.861, -3)
  line L141 (16.861, -3) -> (16.861, -2)
  line L142 (16.861, -2) -> (17.6346, -2)
  line L143 (17.6346, -2) -> (17.6346, -3)
  line L144 (17.6337, -1.0613) -> (16.8602, -1.0613)
  line L145 (16.8602, -1.0613) -> (16.8602, -0.0613)
  line L146 (16.8602, -0.0613) -> (17.6337, -0.0613)
  line L147 (17.6337, -0.0613) -> (17.6337, -1.0613)
  line L148 (17.6337, 1.1028) -> (16.8602, 1.1028)
  line L149 (16.8602, 1.1028) -> (16.8602, 2.1028)
  line L150 (16.8602, 2.1028) -> (17.6337, 2.1028)
  line L151 (17.6337, 2.1028) -> (17.6337, 1.1028)
  line L152 (17.6346, 3) -> (16.861, 3)
  line L153 (16.861, 3) -> (16.861, 4)
  line L154 (16.861, 4) -> (17.6346, 4)
  line L155 (17.6346, 4) -> (17.6346, 3)
  line L156 (17.6346, 5) -> (16.861, 5)
  line L157 (16.861, 5) -> (16.861, 6)
  line L158 (16.861, 6) -> (17.6346, 6)
  line L159 (17.6346, 6) -> (17.6346, 5)
  line L160 (16.861, 8) -> (17.6346, 8)
  line L161 (17.6346, 8) -> (17.6346, 7)
  line L162 (17.6346, 7) -> (16.861, 7)
  line L163 (16.861, 7) -> (16.861, 8)
  line L164 (21, -9) -> (18.5, -9)
  line L165 (18.5, 8) -> (18.5, -9)
  point P0 (0, 0)
extrude "Extrusion8" cut sketch "Sketch8" against normal blind 1 contours L19 L18 L17 L16 L15 L14 L13 L12 L11 L10 L9 L8 L7 L6 L5 L4 L3 L2 L1 L0 | L39 L38 L37 L36 L35 L34 L33 L32 L31 L30 L29 L28 L27 L26 L25 L24 L23 L22 L21 L20 | L59 L58 L57 L56 L55 L54 L53 L52 L51 L50 L49 L48 L47 L46 L45 L44 L43 L42 L41 L40 | L63 L62 L61 L60 | L67 L66 L65 L64 | L71 L70 L69 L68 | L91 L90 L89 L88 L87 L86 L85 L84 L83 L82 L81 L80 L79 L78 L77 L76 L75 L74 L73 L72 | L99 L98 L165 L92
sketch "Sketch9" plane through (0, 0, 2.75) normal (0, 0, 1) x (1, 0, 0)
  line L0 (-9, 6) -> (-9, 5.75) projected
  line L1 (-10, 6) -> (-9, 6) projected
  line L2 (-10, 5) -> (-10, 6) projected
  line L3 (-9.7112, 5) -> (-10, 5) projected
  line L4 (-10, 2) -> (-9.7112, 2) projected
  line L5 (-10, 1) -> (-10, 2) projected
  line L6 (-9, 1) -> (-10, 1) projected
  line L7 (-9, 1.25) -> (-9, 1) projected
  line L8 (-4, 1) -> (-4, 1.25) projected
  line L9 (-3, 1) -> (-4, 1) projected
  line L10 (-3, 2) -> (-3, 1) projected
  line L11 (-3.2888, 2) -> (-3, 2) projected
  line L12 (-3, 5) -> (-3.2888, 5) projected
  line L13 (-3, 6) -> (-3, 5) projected
  line L14 (-4, 6) -> (-3, 6) projected
  line L15 (-4, 5.75) -> (-4, 6) projected
  line L16 (-5, -20.75) -> (-10, -20.75) projected
  line L17 (-5, -21) -> (-5, -20.75) projected
  line L18 (-4, -21) -> (-5, -21) projected
  line L19 (-4, -20) -> (-4, -21) projected
  line L20 (-4.2888, -20) -> (-4, -20) projected
  line L21 (-4.2888, -17) -> (-4.2888, -20) projected
  line L22 (-4, -17) -> (-4.2888, -17) projected
  line L23 (-4, -16) -> (-4, -17) projected
  line L24 (-5, -16) -> (-4, -16) projected
  line L25 (-5, -16.25) -> (-5, -16) projected
  line L26 (-10, -16.25) -> (-5, -16.25) projected
  line L27 (-10, -16) -> (-10, -16.25) projected
  line L28 (-11, -16) -> (-10, -16) projected
  line L29 (-11, -17) -> (-11, -16) projected
  line L30 (-10.7112, -17) -> (-11, -17) projected
  line L31 (-10.7112, -20) -> (-10.7112, -17) projected
  line L32 (-11, -20) -> (-10.7112, -20) projected
  line L33 (-11, -21) -> (-11, -20) projected
  line L34 (-10, -21) -> (-11, -21) projected
  line L35 (-10, -20.75) -> (-10, -21) projected
  circle A0 centre (-7.5, -18.5) radius 1.9686 projected
  line L36 (-5.3467, -12.75) -> (-10.3467, -12.75) projected
  line L37 (-5.3467, -13) -> (-5.3467, -12.75) projected
  line L38 (-4.3467, -13) -> (-5.3467, -13) projected
  line L39 (-4.3467, -12) -> (-4.3467, -13) projected
  line L40 (-4.6355, -12) -> (-4.3467, -12) projected
  line L41 (-4.6355, -9) -> (-4.6355, -12) projected
  line L42 (-4.3467, -9) -> (-4.6355, -9) projected
  line L43 (-4.3467, -8) -> (-4.3467, -9) projected
  line L44 (-5.3467, -8) -> (-4.3467, -8) projected
  line L45 (-5.3467, -8.25) -> (-5.3467, -8) projected
  line L46 (-10.3467, -8.25) -> (-5.3467, -8.25) projected
  line L47 (-10.3467, -8) -> (-10.3467, -8.25) projected
  line L48 (-11.3467, -8) -> (-10.3467, -8) projected
  line L49 (-11.3467, -9) -> (-11.3467, -8) projected
  line L50 (-11.0579, -9) -> (-11.3467, -9) projected
  line L51 (-11.0579, -12) -> (-11.0579, -9) projected
  line L52 (-11.3467, -12) -> (-11.0579, -12) projected
  line L53 (-11.3467, -13) -> (-11.3467, -12) projected
  line L54 (-10.3467, -13) -> (-11.3467, -13) projected
  line L55 (-10.3467, -12.75) -> (-10.3467, -13) projected
  circle A1 centre (-7.8467, -10.5) radius 1.9686 projected
  line L56 (5, -16.25) -> (10, -16.25) projected
  line L57 (5, -16) -> (5, -16.25) projected
  line L58 (4, -16) -> (5, -16) projected
  line L59 (4, -17) -> (4, -16) projected
  line L60 (4.2888, -17) -> (4, -17) projected
  line L61 (4.2888, -20) -> (4.2888, -17) projected
  line L62 (4, -20) -> (4.2888, -20) projected
  line L63 (4, -21) -> (4, -20) projected
  line L64 (5, -21) -> (4, -21) projected
  line L65 (5, -20.75) -> (5, -21) projected
  line L66 (10, -20.75) -> (5, -20.75) projected
  line L67 (10, -21) -> (10, -20.75) projected
  line L68 (11, -21) -> (10, -21) projected
  line L69 (11, -20) -> (11, -21) projected
  line L70 (10.7112, -20) -> (11, -20) projected
  line L71 (10.7112, -17) -> (10.7112, -20) projected
  line L72 (11, -17) -> (10.7112, -17) projected
  line L73 (11, -16) -> (11, -17) projected
  line L74 (10, -16) -> (11, -16) projected
  line L75 (10, -16.25) -> (10, -16) projected
  circle A2 centre (7.5, -18.5) radius 1.9686 projected
  line L76 (-9, 5.75) -> (-4, 5.75) projected
  line L77 (-9, 6) -> (-9, 5.75) projected
  line L78 (-10, 6) -> (-9, 6) projected
  line L79 (-10, 5) -> (-10, 6) projected
  line L80 (-9.7112, 5) -> (-10, 5) projected
  line L81 (-9.7112, 2) -> (-9.7112, 5) projected
  line L82 (-10, 2) -> (-9.7112, 2) projected
  line L83 (-10, 1) -> (-10, 2) projected
  line L84 (-9, 1) -> (-10, 1) projected
  line L85 (-9, 1.25) -> (-9, 1) projected
  line L86 (-4, 1.25) -> (-9, 1.25) projected
  line L87 (-4, 1) -> (-4, 1.25) projected
  line L88 (-3, 1) -> (-4, 1) projected
  line L89 (-3, 2) -> (-3, 1) projected
  line L90 (-3.2888, 2) -> (-3, 2) projected
  line L91 (-3.2888, 5) -> (-3.2888, 2) projected
  line L92 (-3, 5) -> (-3.2888, 5) projected
  line L93 (-3, 6) -> (-3, 5) projected
  line L94 (-4, 6) -> (-3, 6) projected
  line L95 (-4, 5.75) -> (-4, 6) projected
  line L96 (-10, 6) -> (-9, 6) projected
  line L97 (-10, 6) -> (-9, 6)
  line L98 (-9, 6) -> (-9, 5)
  line L99 (-9, 5) -> (-10, 5)
  line L100 (-10, 5) -> (-10, 6)
  line L101 (-4, 6) -> (-4, 5.75) projected
  line L102 (-3, 6) -> (-3, 5) projected
  line L103 (-4, 6) -> (-3, 6)
  line L104 (-3, 6) -> (-3, 5)
  line L105 (-3, 5) -> (-4, 5)
  line L106 (-4, 5) -> (-4, 6)
  line L107 (-3, 1) -> (-4, 1) projected
  line L108 (-3, 2) -> (-4, 2)
  line L109 (-4, 2) -> (-4, 1)
  line L110 (-4, 1) -> (-3, 1)
  line L111 (-3, 1) -> (-3, 2)
  line L112 (-9, 1) -> (-10, 1) projected
  line L113 (-10, 1) -> (-9, 1)
  line L114 (-9, 1) -> (-9, 2)
  line L115 (-9, 2) -> (-10, 2)
  line L116 (-10, 2) -> (-10, 1)
  line L117 (-11.3467, -8) -> (-10.3467, -8) projected
  line L118 (-11.3467, -8) -> (-10.3467, -8)
  line L119 (-10.3467, -8) -> (-10.3467, -9)
  line L120 (-10.3467, -9) -> (-11.3467, -9)
  line L121 (-11.3467, -9) -> (-11.3467, -8)
  line L122 (-4.3467, -8) -> (-4.3467, -9) projected
  line L123 (-4.3467, -8) -> (-5.3467, -8)
  line L124 (-5.3467, -8) -> (-5.3467, -9)
  line L125 (-5.3467, -9) -> (-4.3467, -9)
  line L126 (-4.3467, -9) -> (-4.3467, -8)
  line L127 (-4.3467, -13) -> (-5.3467, -13)
  line L128 (-5.3467, -13) -> (-5.3467, -12)
  line L129 (-5.3467, -12) -> (-4.3467, -12)
  line L130 (-4.3467, -12) -> (-4.3467, -13)
  line L131 (-10.3467, -13) -> (-11.3467, -13) projected
  line L132 (-11.3467, -13) -> (-10.3467, -13)
  line L133 (-10.3467, -13) -> (-10.3467, -12)
  line L134 (-10.3467, -12) -> (-11.3467, -12)
  line L135 (-11.3467, -12) -> (-11.3467, -13)
  line L136 (-11, -16) -> (-10, -16)
  line L137 (-10, -16) -> (-10, -17)
  line L138 (-10, -17) -> (-11, -17)
  line L139 (-11, -17) -> (-11, -16)
  line L140 (-4, -16) -> (-5, -16)
  line L141 (-5, -16) -> (-5, -17)
  line L142 (-5, -17) -> (-4, -17)
  line L143 (-4, -17) -> (-4, -16)
  line L144 (-4, -21) -> (-5, -21)
  line L145 (-5, -21) -> (-5, -20)
  line L146 (-5, -20) -> (-4, -20)
  line L147 (-4, -20) -> (-4, -21)
  line L148 (-11, -21) -> (-10, -21)
  line L149 (-10, -21) -> (-10, -20)
  line L150 (-10, -20) -> (-11, -20)
  line L151 (-11, -20) -> (-11, -21)
  line L152 (4, -16) -> (5, -16)
  line L153 (5, -16) -> (5, -17)
  line L154 (5, -17) -> (4, -17)
  line L155 (4, -17) -> (4, -16)
  line L156 (11, -16) -> (10, -16)
  line L157 (10, -16) -> (10, -17)
  line L158 (10, -17) -> (11, -17)
  line L159 (11, -17) -> (11, -16)
  line L160 (11, -21) -> (10, -21)
  line L161 (10, -21) -> (10, -20)
  line L162 (10, -20) -> (11, -20)
  line L163 (11, -20) -> (11, -21)
  line L164 (4, -21) -> (5, -21)
  line L165 (5, -21) -> (5, -20)
  line L166 (5, -20) -> (4, -20)
  line L167 (4, -20) -> (4, -21)
  point P0 (0, 0)
  constraints: 128 end point, 32 parallel, 16 horizontal, 16 perpendicular, 8 point on line
extrude "Extrusion9" cut sketch "Sketch9" against normal blind 1 contours L0 L98 L99 L3 L2 L1 | L15 L14 L13 L12 L105 L106 | L115 L114 L7 L6 L5 L4 | L11 L10 L9 L8 L109 L108 | L145 L146 L20 L19 L18 L17 | L35 L34 L33 L32 L150 L149 | L142 L141 L25 L24 L23 L22 | L30 L29 L28 L27 L137 L138 | L128 L129 L40 L39 L38 L37 | L55 L54 L53 L52 L134 L133 | L125 L124 L45 L44 L43 L42 | L50 L49 L48 L47 L119 L120 | L153 L154 L60 L59 L58 L57 | L75 L74 L73 L72 L158 L157 | L166 L165 L65 L64 L63 L62 | L70 L69 L68 L67 L161 L162
fillet "Fillet1" radius 0.25 5 edges at (-9.6897, -10.5, 3) (-9.3436, -18.5, 3) (5.6564, -18.5, 3) (8.5453, 12.5, 3) (-10.392, 12.5, 3)